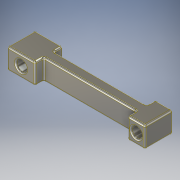
# Autodesk Inventor part: Connecting Rod
Saved by Autodesk Inventor 2017 (Build 210142000, 142)
## iProperties
Created: 2020-01-12
Part Number: Connecting Rod
Material: Silver
Document SubType Name: Modeling
Designer: Admin
Density: 10.49 g/cm^3
Appearance: Silver
Mass: 5.11131 g
Surface Area: 6.63602 cm^2
Volume: 0.487255 cm^3
Author: Admin
Autodesk Inventor part; units mm, degrees
ref_plane "YZ Plane" through (0, 0, 0) normal (1, 0, 0) x (0, 1, 0)
ref_plane "XZ Plane" through (0, 0, 0) normal (0, 1, 0) x (-1, 0, 0)
ref_plane "XY Plane" through (0, 0, 0) normal (0, 0, 1) x (1, 0, 0)
sketch "Sketch1" plane through (0, 0, 0) normal (0, 1, 0) x (-1, 0, 0)
  line L0 (15.6766, -3.175) -> (9.3266, -3.175)
  line L1 (9.3266, -3.175) -> (9.3266, 3.175)
  line L2 (9.3266, 3.175) -> (15.6766, 3.175)
  line L3 (15.6766, 3.175) -> (15.6766, -3.175)
  line L4 (-11.7078, -3.175) -> (-15.6766, -3.175)
  line L5 (-15.6766, -3.175) -> (-15.6766, 3.175)
  line L6 (-15.6766, 3.175) -> (-11.7078, 3.175)
  line L7 (-11.7078, 3.175) -> (-11.7078, -3.175)
  line L8 (9.3266, -1.1906) -> (-11.7078, -1.1906)
  line L9 (-11.7078, -1.1906) -> (-11.7078, 1.1906)
  line L10 (-11.7078, 1.1906) -> (9.3266, 1.1906)
  line L11 (9.3266, 1.1906) -> (9.3266, -1.1906)
  point P0 (0, 0)
  dimension "d0" = 6.35
  dimension "d1" = 6.35
  dimension "d2" = 3.9688
  dimension "d3" = 6.35
  dimension "d4" = 3.175
  dimension "d5" = 3.175
  dimension "d6" = 31.3531
  dimension "d7" = 9.3266
  dimension "d8" = 2.3813
  dimension "d9" = 1.9844
  constraints: 24 end point, 6 parallel, 3 horizontal, 3 perpendicular, 2 point on line
  measures "d0" distance of L1.end L2.end
  measures "d1" distance of L2.end L0.start
  measures "d2" distance of L5.end L6.end
  measures "d3" distance of L4.end L5.end
  measures "d4" distance from line of point (0, 0) L0
  measures "d5" distance from line of point (0, 0) L4
  measures "d6" distance between parallel lines of L5 L3
  measures "d7" distance from line of point (0, 0) L1
  measures "d8" distance between parallel lines of L10 L8
  measures "d9" distance between parallel lines of L10 L2
extrude "Extrusion1" add sketch "Sketch1" along normal mid plane 4.7625
sketch "Sketch2" plane through (-15.6766, 2.3813, 3.175) normal (0, 0, 1) x (1, 0, 0)
  circle A0 centre (3.175, -2.3813) radius 1.1906
  line L0 (6.35, -4.7625) -> (6.35, 0) projected
  circle A1 centre (29.3688, -2.3813) radius 1.1906
  line L1 (31.3531, -4.7625) -> (31.3531, 0) projected
  point P0 (15.6766, -2.3813)
  dimension "d12" = 2.3813
  dimension "d13" = 3.175
  dimension "d14" = 0
  dimension "d15" = 2.3813
  dimension "d16" = 0
  dimension "d17" = 1.9844
  constraints: 2 centre point
  measures "d12" diameter of A0
  measures "d13" distance from line of L0 A0.centre
  measures "d14" vertical distance of point (15.677, -2.381) A0.centre
  measures "d15" diameter of A1
  measures "d16" vertical distance of point (15.677, -2.381) A1.centre
  measures "d17" distance from line of L1 A1.centre
extrude "Extrusion2" cut sketch "Sketch2" against normal blind 6.35
fillet "Fillet1" radius 0.3969 4 edges at (-9.3266, 0, 1.1906) (-9.3266, 0, -1.1906) (11.7078, 0, -1.1906) (11.7078, 0, 1.1906)
fillet "Fillet2" radius 0.3969 24 edges at (-9.2103, -2.3813, 1.3069) (1.1906, -2.3813, 1.1906) (11.5916, -2.3813, 1.3069) (11.7078, -2.3813, 2.3812) (-9.3266, -2.3813, 2.3813) (-9.2103, -2.3813, -1.3069) (1.1906, -2.3813, -1.1906) (11.5916, -2.3813, -1.3069) (11.7078, -2.3813, -2.3813) (-9.3266, -2.3813, -2.3812) (-9.2103, 2.3813, -1.3069) (1.1906, 2.3813, -1.1906) (11.5916, 2.3813, -1.3069) (11.7078, 2.3813, -2.3813) (-9.3266, 2.3813, -2.3812) (-9.2103, 2.3813, 1.3069) (1.1906, 2.3813, 1.1906) (11.5916, 2.3813, 1.3069) (11.7078, 2.3813, 2.3812) (-9.3266, 2.3813, 2.3813) (15.6766, 0, -3.175) (15.6766, 0, 3.175) (-15.6766, 0, 3.175) (-15.6766, 0, -3.175)
fillet "Fillet3" radius 0.3969 32 edges at (-9.3266, 0, -3.175) (-9.4428, 2.265, -3.175) (-12.5016, 2.3813, -3.175) (-15.5603, 2.3813, -3.0588) (-15.6766, 2.3813, 0) (-15.5603, 2.3813, 3.0588) (-12.5016, 2.3813, 3.175) (-9.4428, 2.265, 3.175) (-9.3266, 0, 3.175) (-9.4428, -2.265, 3.175) (-12.5016, -2.3813, 3.175) (-15.5603, -2.3813, 3.0588) (-15.6766, -2.3813, 0) (-15.5603, -2.3813, -3.0588) (-12.5016, -2.3813, -3.175) (-9.4428, -2.265, -3.175) (11.8241, 2.265, -3.175) (13.6922, 2.3813, -3.175) (15.5603, 2.3813, -3.0588) (15.6766, 2.3813, 0) (15.5603, 2.3813, 3.0588) (13.6922, 2.3813, 3.175) (11.8241, 2.265, 3.175) (11.7078, 0, 3.175) (11.8241, -2.265, 3.175) (13.6922, -2.3813, 3.175) (15.5603, -2.3813, 3.0588) (15.6766, -2.3813, 0) (15.5603, -2.3813, -3.0588) (13.6922, -2.3813, -3.175) (11.8241, -2.265, -3.175) (11.7078, 0, -3.175)
fillet "Fillet4" radius 0.3175 4 edges at (-13.6922, 0, 3.175) (-13.6922, 0, -3.175) (12.5016, 0, 3.175) (12.5016, 0, -3.175)
body "Solid1"
